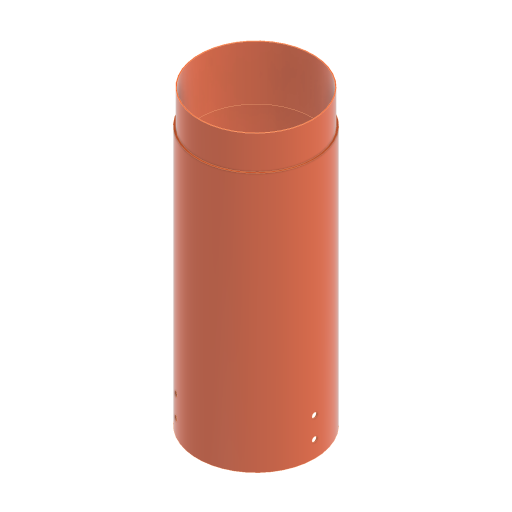
# Autodesk Inventor part: Engine skin
Saved by Autodesk Inventor 2024 (Build 280153000, 153)
## iProperties
Created: 2023-12-30
Part Number: Engine skin
Material: Plastic, Opaque White
Document SubType Name: Modeling
Designer: Jamie
Density: 0.952 g/cm^3
Appearance: Smooth - Light Orange
Author: Jamie
Autodesk Inventor part; units mm, degrees
ref_plane "XZ Plane" through (0, 0, 0) normal (0, 1, 0) x (-1, 0, 0)
sketch "Sketch1" plane through (0, 0, 0) normal (0, 1, 0) x (-1, 0, 0)
  circle A0 centre (0, 0) radius 35
  circle A1 centre (0, 0) radius 34.5
  dimension "d0" = 70
  dimension "d1" = 69
  constraints: 2 centre point, 2 coincident
  measures "d0" diameter of A0
  measures "d1" diameter of A1
extrude "Extrusion1" add sketch "Sketch1" along normal blind 155
ref_plane "Work Plane2" through (35, 0, 0) normal (1, 0, 0) x (0, 1, 0)
sketch "Sketch4" plane through (35, 0, 0) normal (1, 0, 0) x (0, 1, 0)
  line L0 (155, -35) -> (155, 35) projected
  point P0 (0, 0)
  point P1 (10, 0)
  dimension "d48" = 10
  measures "d48" distance of point (0, 0) point (10, 0)
hole "Hole2" at (35, 10, 0) direction (-1, 0, 0) diameter 3 depth 8 tip angle 118
sketch "Sketch5" plane through (0, 155, 0) normal (0, 1, 0) x (1, 0, 0)
  circle A0 centre (0, 0) radius 34
  circle A1 centre (0, 0) radius 33.5
  dimension "d44" = 68
  dimension "d45" = 67
  constraints: 2 centre point, 2 coincident
  measures "d44" diameter of A0
  measures "d45" diameter of A1
extrude "Extrusion3" add sketch "Sketch5" along normal blind 20
sketch "Sketch6" plane through (0, 155, 0) normal (0, -1, 0) x (1, 0, 0)
  circle A0 centre (0, 0) radius 33.5
  circle A1 centre (0, 0) radius 34.5 projected
  circle A2 centre (0, 0) radius 35
  constraints: 2 centre point, 2 coincident
extrude "Extrusion4" add sketch "Sketch6" along normal blind 12.5 contours A1
ref_plane "Work Plane4" through (34, 0, 0) normal (1, 0, 0) x (0, 1, 0)
pattern_circular "Circular Pattern2" count 3 over 360 about axis through (0, 0, 0) along (0, 1, 0) of "Hole2"
sketch "Sketch10" plane through (35, 0, 0) normal (1, 0, 0) x (0, 1, 0)
  point P0 (0, 0)
  point P1 (22.5, 0)
  dimension "d82" = 22.5
  measures "d82" distance of point (0, 0) point (22.5, 0)
hole "Hole6" at (35, 22.5, 0) direction (-1, 0, 0) diameter 3 depth 8 tip angle 118
pattern_circular "Circular Pattern3" count 3 over 360 about axis through (0, 0, 0) along (0, 1, 0) of "Hole6"
body "Solid1"
